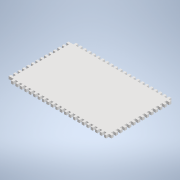
# Autodesk Inventor part: top1
Saved by Autodesk Inventor 2022 (Build 260153000, 153)
## iProperties
Created: 2023-05-26
Part Number: top1
Material: Типовые
Document SubType Name: Modeling
Designer: korsh624
Density: 1 g/cm^3
Appearance: По умолчанию
Author: korsh624
Autodesk Inventor part; units mm, degrees
ref_plane "YZ Plane" through (0, 0, 0) normal (1, 0, 0) x (0, 1, 0)
ref_plane "XZ Plane" through (0, 0, 0) normal (0, 1, 0) x (-1, 0, 0)
ref_plane "XY Plane" through (0, 0, 0) normal (0, 0, 1) x (1, 0, 0)
sketch "Эскиз1" plane through (0, 0, 0) normal (0, 1, 0) x (-1, 0, 0)
  line L0 (-19.1413, -144.0029) -> (200.8587, -144.0029)
  line L1 (200.8587, -144.0029) -> (200.8587, -9.0029)
  line L2 (200.8587, -9.0029) -> (-19.1413, -9.0029)
  line L3 (-19.1413, -9.0029) -> (-19.1413, -144.0029)
  line L4 (-19.1413, -144.0029) -> (-25.1413, -144.0029)
  line L5 (-25.1413, -144.0029) -> (-25.1413, -139.0029)
  line L6 (-25.1413, -139.0029) -> (-19.1413, -139.0029)
  line L7 (-19.1413, -139.0029) -> (-19.1413, -144.0029)
  line L8 (-19.1413, -134.0029) -> (-25.1413, -134.0029)
  line L9 (-25.1413, -134.0029) -> (-25.1413, -129.0029)
  line L10 (-25.1413, -129.0029) -> (-19.1413, -129.0029)
  line L11 (-19.1413, -129.0029) -> (-19.1413, -134.0029)
  line L12 (-19.1413, -124.0029) -> (-25.1413, -124.0029)
  line L13 (-25.1413, -124.0029) -> (-25.1413, -119.0029)
  line L14 (-25.1413, -119.0029) -> (-19.1413, -119.0029)
  line L15 (-19.1413, -119.0029) -> (-19.1413, -124.0029)
  line L16 (-19.1413, -114.0029) -> (-25.1413, -114.0029)
  line L17 (-25.1413, -114.0029) -> (-25.1413, -109.0029)
  line L18 (-25.1413, -109.0029) -> (-19.1413, -109.0029)
  line L19 (-19.1413, -109.0029) -> (-19.1413, -114.0029)
  line L20 (-19.1413, -104.0029) -> (-25.1413, -104.0029)
  line L21 (-25.1413, -104.0029) -> (-25.1413, -99.0029)
  line L22 (-25.1413, -99.0029) -> (-19.1413, -99.0029)
  line L23 (-19.1413, -99.0029) -> (-19.1413, -104.0029)
  line L24 (-19.1413, -94.0029) -> (-25.1413, -94.0029)
  line L25 (-25.1413, -94.0029) -> (-25.1413, -89.0029)
  line L26 (-25.1413, -89.0029) -> (-19.1413, -89.0029)
  line L27 (-19.1413, -89.0029) -> (-19.1413, -94.0029)
  line L28 (-19.1413, -84.0029) -> (-25.1413, -84.0029)
  line L29 (-25.1413, -84.0029) -> (-25.1413, -79.0029)
  line L30 (-25.1413, -79.0029) -> (-19.1413, -79.0029)
  line L31 (-19.1413, -79.0029) -> (-19.1413, -84.0029)
  line L32 (-19.1413, -74.0029) -> (-25.1413, -74.0029)
  line L33 (-25.1413, -74.0029) -> (-25.1413, -69.0029)
  line L34 (-25.1413, -69.0029) -> (-19.1413, -69.0029)
  line L35 (-19.1413, -69.0029) -> (-19.1413, -74.0029)
  line L36 (-19.1413, -64.0029) -> (-25.1413, -64.0029)
  line L37 (-25.1413, -64.0029) -> (-25.1413, -59.0029)
  line L38 (-25.1413, -59.0029) -> (-19.1413, -59.0029)
  line L39 (-19.1413, -59.0029) -> (-19.1413, -64.0029)
  line L40 (-19.1413, -54.0029) -> (-25.1413, -54.0029)
  line L41 (-25.1413, -54.0029) -> (-25.1413, -49.0029)
  line L42 (-25.1413, -49.0029) -> (-19.1413, -49.0029)
  line L43 (-19.1413, -49.0029) -> (-19.1413, -54.0029)
  line L44 (-19.1413, -44.0029) -> (-25.1413, -44.0029)
  line L45 (-25.1413, -44.0029) -> (-25.1413, -39.0029)
  line L46 (-25.1413, -39.0029) -> (-19.1413, -39.0029)
  line L47 (-19.1413, -39.0029) -> (-19.1413, -44.0029)
  line L48 (-19.1413, -34.0029) -> (-25.1413, -34.0029)
  line L49 (-25.1413, -34.0029) -> (-25.1413, -29.0029)
  line L50 (-25.1413, -29.0029) -> (-19.1413, -29.0029)
  line L51 (-19.1413, -29.0029) -> (-19.1413, -34.0029)
  line L52 (-19.1413, -24.0029) -> (-25.1413, -24.0029)
  line L53 (-25.1413, -24.0029) -> (-25.1413, -19.0029)
  line L54 (-25.1413, -19.0029) -> (-19.1413, -19.0029)
  line L55 (-19.1413, -19.0029) -> (-19.1413, -24.0029)
  line L56 (-19.1413, -14.0029) -> (-25.1413, -14.0029)
  line L57 (-25.1413, -14.0029) -> (-25.1413, -9.0029)
  line L58 (-25.1413, -9.0029) -> (-19.1413, -9.0029)
  line L59 (-19.1413, -9.0029) -> (-19.1413, -14.0029)
  line L60 (90.8587, -185.2941) -> (90.8587, 117.247) construction
  line L61 (214.3275, -76.5029) -> (-83.7426, -76.5029) construction
  line L62 (-19.1413, -9.0029) -> (-14.1413, -9.0029)
  line L63 (-14.1413, -9.0029) -> (-14.1413, -3.0029)
  line L64 (-14.1413, -3.0029) -> (-19.1413, -3.0029)
  line L65 (-19.1413, -3.0029) -> (-19.1413, -9.0029)
  line L66 (224.3275, -76.5029) -> (-73.7426, -76.5029) construction
  line L67 (-9.1413, -3.0029) -> (-9.1413, -9.0029)
  line L68 (-4.1413, -9.0029) -> (-4.1413, -3.0029)
  line L69 (-4.1413, -3.0029) -> (-9.1413, -3.0029)
  line L70 (234.3275, -76.5029) -> (-63.7426, -76.5029) construction
  line L71 (0.8587, -3.0029) -> (0.8587, -9.0029)
  line L72 (5.8587, -9.0029) -> (5.8587, -3.0029)
  line L73 (5.8587, -3.0029) -> (0.8587, -3.0029)
  line L74 (244.3275, -76.5029) -> (-53.7426, -76.5029) construction
  line L75 (10.8587, -3.0029) -> (10.8587, -9.0029)
  line L76 (15.8587, -9.0029) -> (15.8587, -3.0029)
  line L77 (15.8587, -3.0029) -> (10.8587, -3.0029)
  line L78 (254.3275, -76.5029) -> (-43.7426, -76.5029) construction
  line L79 (20.8587, -3.0029) -> (20.8587, -9.0029)
  line L80 (25.8587, -9.0029) -> (25.8587, -3.0029)
  line L81 (25.8587, -3.0029) -> (20.8587, -3.0029)
  line L82 (264.3275, -76.5029) -> (-33.7426, -76.5029) construction
  line L83 (30.8587, -3.0029) -> (30.8587, -9.0029)
  line L84 (35.8587, -9.0029) -> (35.8587, -3.0029)
  line L85 (35.8587, -3.0029) -> (30.8587, -3.0029)
  line L86 (274.3275, -76.5029) -> (-23.7426, -76.5029) construction
  line L87 (40.8587, -3.0029) -> (40.8587, -9.0029)
  line L88 (45.8587, -9.0029) -> (45.8587, -3.0029)
  line L89 (45.8587, -3.0029) -> (40.8587, -3.0029)
  line L90 (284.3275, -76.5029) -> (-13.7426, -76.5029) construction
  line L91 (50.8587, -3.0029) -> (50.8587, -9.0029)
  line L92 (55.8587, -9.0029) -> (55.8587, -3.0029)
  line L93 (55.8587, -3.0029) -> (50.8587, -3.0029)
  line L94 (294.3275, -76.5029) -> (-3.7426, -76.5029) construction
  line L95 (60.8587, -3.0029) -> (60.8587, -9.0029)
  line L96 (65.8587, -9.0029) -> (65.8587, -3.0029)
  line L97 (65.8587, -3.0029) -> (60.8587, -3.0029)
  line L98 (304.3275, -76.5029) -> (6.2574, -76.5029) construction
  line L99 (70.8587, -3.0029) -> (70.8587, -9.0029)
  line L100 (75.8587, -9.0029) -> (75.8587, -3.0029)
  line L101 (75.8587, -3.0029) -> (70.8587, -3.0029)
  line L102 (314.3275, -76.5029) -> (16.2574, -76.5029) construction
  line L103 (80.8587, -3.0029) -> (80.8587, -9.0029)
  line L104 (85.8587, -9.0029) -> (85.8587, -3.0029)
  line L105 (85.8587, -3.0029) -> (80.8587, -3.0029)
  line L106 (324.3275, -76.5029) -> (26.2574, -76.5029) construction
  line L107 (90.8587, -3.0029) -> (90.8587, -9.0029)
  line L108 (95.8587, -9.0029) -> (95.8587, -3.0029)
  line L109 (95.8587, -3.0029) -> (90.8587, -3.0029)
  line L110 (334.3275, -76.5029) -> (36.2574, -76.5029) construction
  line L111 (100.8587, -3.0029) -> (100.8587, -9.0029)
  line L112 (105.8587, -9.0029) -> (105.8587, -3.0029)
  line L113 (105.8587, -3.0029) -> (100.8587, -3.0029)
  line L114 (344.3275, -76.5029) -> (46.2574, -76.5029) construction
  line L115 (110.8587, -3.0029) -> (110.8587, -9.0029)
  line L116 (115.8587, -9.0029) -> (115.8587, -3.0029)
  line L117 (115.8587, -3.0029) -> (110.8587, -3.0029)
  line L118 (354.3275, -76.5029) -> (56.2574, -76.5029) construction
  line L119 (120.8587, -3.0029) -> (120.8587, -9.0029)
  line L120 (125.8587, -9.0029) -> (125.8587, -3.0029)
  line L121 (125.8587, -3.0029) -> (120.8587, -3.0029)
  line L122 (364.3275, -76.5029) -> (66.2574, -76.5029) construction
  line L123 (130.8587, -3.0029) -> (130.8587, -9.0029)
  line L124 (135.8587, -9.0029) -> (135.8587, -3.0029)
  line L125 (135.8587, -3.0029) -> (130.8587, -3.0029)
  line L126 (374.3275, -76.5029) -> (76.2574, -76.5029) construction
  line L127 (140.8587, -3.0029) -> (140.8587, -9.0029)
  line L128 (145.8587, -9.0029) -> (145.8587, -3.0029)
  line L129 (145.8587, -3.0029) -> (140.8587, -3.0029)
  line L130 (384.3275, -76.5029) -> (86.2574, -76.5029) construction
  line L131 (150.8587, -3.0029) -> (150.8587, -9.0029)
  line L132 (155.8587, -9.0029) -> (155.8587, -3.0029)
  line L133 (155.8587, -3.0029) -> (150.8587, -3.0029)
  line L134 (394.3275, -76.5029) -> (96.2574, -76.5029) construction
  line L135 (160.8587, -3.0029) -> (160.8587, -9.0029)
  line L136 (165.8587, -9.0029) -> (165.8587, -3.0029)
  line L137 (165.8587, -3.0029) -> (160.8587, -3.0029)
  line L138 (404.3275, -76.5029) -> (106.2574, -76.5029) construction
  line L139 (170.8587, -3.0029) -> (170.8587, -9.0029)
  line L140 (175.8587, -9.0029) -> (175.8587, -3.0029)
  line L141 (175.8587, -3.0029) -> (170.8587, -3.0029)
  line L142 (414.3275, -76.5029) -> (116.2574, -76.5029) construction
  line L143 (180.8587, -3.0029) -> (180.8587, -9.0029)
  line L144 (185.8587, -9.0029) -> (185.8587, -3.0029)
  line L145 (185.8587, -3.0029) -> (180.8587, -3.0029)
  line L146 (424.3275, -76.5029) -> (126.2574, -76.5029) construction
  line L147 (190.8587, -3.0029) -> (190.8587, -9.0029)
  line L148 (195.8587, -9.0029) -> (195.8587, -3.0029)
  line L149 (195.8587, -3.0029) -> (190.8587, -3.0029)
  line L150 (200.8587, -144.0029) -> (206.8587, -144.0029)
  line L151 (206.8587, -144.0029) -> (206.8587, -139.0029)
  line L152 (206.8587, -139.0029) -> (200.8587, -139.0029)
  line L153 (200.8587, -139.0029) -> (200.8587, -144.0029)
  line L154 (200.8587, -134.0029) -> (206.8587, -134.0029)
  line L155 (206.8587, -134.0029) -> (206.8587, -129.0029)
  line L156 (206.8587, -129.0029) -> (200.8587, -129.0029)
  line L157 (200.8587, -129.0029) -> (200.8587, -134.0029)
  line L158 (200.8587, -124.0029) -> (206.8587, -124.0029)
  line L159 (206.8587, -124.0029) -> (206.8587, -119.0029)
  line L160 (206.8587, -119.0029) -> (200.8587, -119.0029)
  line L161 (200.8587, -119.0029) -> (200.8587, -124.0029)
  line L162 (200.8587, -114.0029) -> (206.8587, -114.0029)
  line L163 (206.8587, -114.0029) -> (206.8587, -109.0029)
  line L164 (206.8587, -109.0029) -> (200.8587, -109.0029)
  line L165 (200.8587, -109.0029) -> (200.8587, -114.0029)
  line L166 (200.8587, -104.0029) -> (206.8587, -104.0029)
  line L167 (206.8587, -104.0029) -> (206.8587, -99.0029)
  line L168 (206.8587, -99.0029) -> (200.8587, -99.0029)
  line L169 (200.8587, -99.0029) -> (200.8587, -104.0029)
  line L170 (200.8587, -94.0029) -> (206.8587, -94.0029)
  line L171 (206.8587, -94.0029) -> (206.8587, -89.0029)
  line L172 (206.8587, -89.0029) -> (200.8587, -89.0029)
  line L173 (200.8587, -89.0029) -> (200.8587, -94.0029)
  line L174 (200.8587, -84.0029) -> (206.8587, -84.0029)
  line L175 (206.8587, -84.0029) -> (206.8587, -79.0029)
  line L176 (206.8587, -79.0029) -> (200.8587, -79.0029)
  line L177 (200.8587, -79.0029) -> (200.8587, -84.0029)
  line L178 (200.8587, -74.0029) -> (206.8587, -74.0029)
  line L179 (206.8587, -74.0029) -> (206.8587, -69.0029)
  line L180 (206.8587, -69.0029) -> (200.8587, -69.0029)
  line L181 (200.8587, -69.0029) -> (200.8587, -74.0029)
  line L182 (200.8587, -64.0029) -> (206.8587, -64.0029)
  line L183 (206.8587, -64.0029) -> (206.8587, -59.0029)
  line L184 (206.8587, -59.0029) -> (200.8587, -59.0029)
  line L185 (200.8587, -59.0029) -> (200.8587, -64.0029)
  line L186 (200.8587, -54.0029) -> (206.8587, -54.0029)
  line L187 (206.8587, -54.0029) -> (206.8587, -49.0029)
  line L188 (206.8587, -49.0029) -> (200.8587, -49.0029)
  line L189 (200.8587, -49.0029) -> (200.8587, -54.0029)
  line L190 (200.8587, -44.0029) -> (206.8587, -44.0029)
  line L191 (206.8587, -44.0029) -> (206.8587, -39.0029)
  line L192 (206.8587, -39.0029) -> (200.8587, -39.0029)
  line L193 (200.8587, -39.0029) -> (200.8587, -44.0029)
  line L194 (200.8587, -34.0029) -> (206.8587, -34.0029)
  line L195 (206.8587, -34.0029) -> (206.8587, -29.0029)
  line L196 (206.8587, -29.0029) -> (200.8587, -29.0029)
  line L197 (200.8587, -29.0029) -> (200.8587, -34.0029)
  line L198 (200.8587, -24.0029) -> (206.8587, -24.0029)
  line L199 (206.8587, -24.0029) -> (206.8587, -19.0029)
  line L200 (206.8587, -19.0029) -> (200.8587, -19.0029)
  line L201 (200.8587, -19.0029) -> (200.8587, -24.0029)
  line L202 (200.8587, -14.0029) -> (206.8587, -14.0029)
  line L203 (206.8587, -14.0029) -> (206.8587, -9.0029)
  line L204 (206.8587, -9.0029) -> (200.8587, -9.0029)
  line L205 (200.8587, -9.0029) -> (200.8587, -14.0029)
  line L206 (90.8587, 32.2883) -> (90.8587, -270.2529) construction
  line L207 (-14.1413, -144.0029) -> (-14.1413, -150.0029)
  line L208 (-14.1413, -150.0029) -> (-19.1413, -150.0029)
  line L209 (-19.1413, -150.0029) -> (-19.1413, -144.0029)
  line L210 (-9.1413, -150.0029) -> (-9.1413, -144.0029)
  line L211 (-4.1413, -144.0029) -> (-4.1413, -150.0029)
  line L212 (-4.1413, -150.0029) -> (-9.1413, -150.0029)
  line L213 (0.8587, -150.0029) -> (0.8587, -144.0029)
  line L214 (5.8587, -144.0029) -> (5.8587, -150.0029)
  line L215 (5.8587, -150.0029) -> (0.8587, -150.0029)
  line L216 (10.8587, -150.0029) -> (10.8587, -144.0029)
  line L217 (15.8587, -144.0029) -> (15.8587, -150.0029)
  line L218 (15.8587, -150.0029) -> (10.8587, -150.0029)
  line L219 (20.8587, -150.0029) -> (20.8587, -144.0029)
  line L220 (25.8587, -144.0029) -> (25.8587, -150.0029)
  line L221 (25.8587, -150.0029) -> (20.8587, -150.0029)
  line L222 (30.8587, -150.0029) -> (30.8587, -144.0029)
  line L223 (35.8587, -144.0029) -> (35.8587, -150.0029)
  line L224 (35.8587, -150.0029) -> (30.8587, -150.0029)
  line L225 (40.8587, -150.0029) -> (40.8587, -144.0029)
  line L226 (45.8587, -144.0029) -> (45.8587, -150.0029)
  line L227 (45.8587, -150.0029) -> (40.8587, -150.0029)
  line L228 (50.8587, -150.0029) -> (50.8587, -144.0029)
  line L229 (55.8587, -144.0029) -> (55.8587, -150.0029)
  line L230 (55.8587, -150.0029) -> (50.8587, -150.0029)
  line L231 (60.8587, -150.0029) -> (60.8587, -144.0029)
  line L232 (65.8587, -144.0029) -> (65.8587, -150.0029)
  line L233 (65.8587, -150.0029) -> (60.8587, -150.0029)
  line L234 (70.8587, -150.0029) -> (70.8587, -144.0029)
  line L235 (75.8587, -144.0029) -> (75.8587, -150.0029)
  line L236 (75.8587, -150.0029) -> (70.8587, -150.0029)
  line L237 (80.8587, -150.0029) -> (80.8587, -144.0029)
  line L238 (85.8587, -144.0029) -> (85.8587, -150.0029)
  line L239 (85.8587, -150.0029) -> (80.8587, -150.0029)
  line L240 (90.8587, -150.0029) -> (90.8587, -144.0029)
  line L241 (95.8587, -144.0029) -> (95.8587, -150.0029)
  line L242 (95.8587, -150.0029) -> (90.8587, -150.0029)
  line L243 (100.8587, -150.0029) -> (100.8587, -144.0029)
  line L244 (105.8587, -144.0029) -> (105.8587, -150.0029)
  line L245 (105.8587, -150.0029) -> (100.8587, -150.0029)
  line L246 (110.8587, -150.0029) -> (110.8587, -144.0029)
  line L247 (115.8587, -144.0029) -> (115.8587, -150.0029)
  line L248 (115.8587, -150.0029) -> (110.8587, -150.0029)
  line L249 (120.8587, -150.0029) -> (120.8587, -144.0029)
  line L250 (125.8587, -144.0029) -> (125.8587, -150.0029)
  line L251 (125.8587, -150.0029) -> (120.8587, -150.0029)
  line L252 (130.8587, -150.0029) -> (130.8587, -144.0029)
  line L253 (135.8587, -144.0029) -> (135.8587, -150.0029)
  line L254 (135.8587, -150.0029) -> (130.8587, -150.0029)
  line L255 (140.8587, -150.0029) -> (140.8587, -144.0029)
  line L256 (145.8587, -144.0029) -> (145.8587, -150.0029)
  line L257 (145.8587, -150.0029) -> (140.8587, -150.0029)
  line L258 (150.8587, -150.0029) -> (150.8587, -144.0029)
  line L259 (155.8587, -144.0029) -> (155.8587, -150.0029)
  line L260 (155.8587, -150.0029) -> (150.8587, -150.0029)
  line L261 (160.8587, -150.0029) -> (160.8587, -144.0029)
  line L262 (165.8587, -144.0029) -> (165.8587, -150.0029)
  line L263 (165.8587, -150.0029) -> (160.8587, -150.0029)
  line L264 (170.8587, -150.0029) -> (170.8587, -144.0029)
  line L265 (175.8587, -144.0029) -> (175.8587, -150.0029)
  line L266 (175.8587, -150.0029) -> (170.8587, -150.0029)
  line L267 (180.8587, -150.0029) -> (180.8587, -144.0029)
  line L268 (185.8587, -144.0029) -> (185.8587, -150.0029)
  line L269 (185.8587, -150.0029) -> (180.8587, -150.0029)
  line L270 (190.8587, -150.0029) -> (190.8587, -144.0029)
  line L271 (195.8587, -144.0029) -> (195.8587, -150.0029)
  line L272 (195.8587, -150.0029) -> (190.8587, -150.0029)
  point P0 (0, 0)
  point P1 (215.4601, -76.5029)
  point P2 (205.4601, -76.5029)
  point P3 (0, -153.0059)
  dimension "d0" = 220
  dimension "d1" = 135
  dimension "d2" = 6
  dimension "d3" = 5
  dimension "d6" = 10
  dimension "d11" = 67.5
  dimension "d12" = 5
  dimension "d13" = 6
  dimension "d16" = 10
  constraints: 538 end point, 148 symmetric about line, 126 horizontal alignment, 72 parallel, 68 collinear, 52 vertical alignment, 3 horizontal, 2 perpendicular, 1 vertical, 12 other
  measures "d0" distance of point (200.859, -9.003) point (-19.141, -9.003)
  measures "d1" distance of point (-19.141, -9.003) L4.start
  measures "d2" distance of L5.end L6.end
  measures "d3" distance of L4.end L5.end
  measures "d6" distance of L4.start L8.start
  measures "d12" distance of L64.end L63.end
  measures "d13" distance of L63.end L62.end
  measures "d16" distance of L61.start L66.start
extrude "Выдавливание1" add sketch "Эскиз1" along normal blind 6
equation "\"d11\" = 0.5 * d1"
